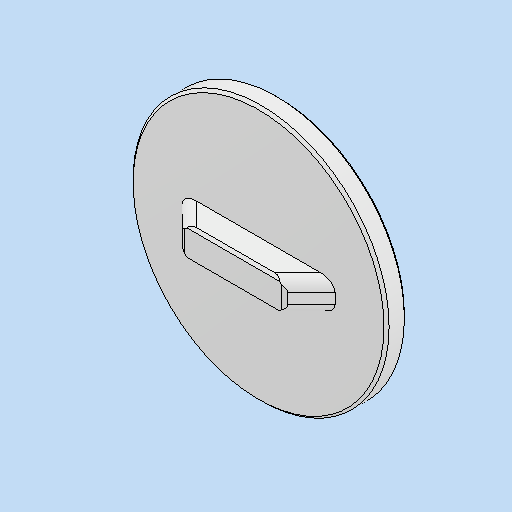
# Autodesk Inventor part: Sensor-Cap
Saved by Autodesk Inventor 2025 (Build 290162000, 162)
## iProperties
Created: 2025-02-18
Part Number: Sensor-Cap
Material: ABS Plastic
Document SubType Name: Modeling
Designer: kuzmin
Density: 1.06 g/cm^3
Appearance: Smooth - White
Author: kuzmin
Autodesk Inventor part; units mm, degrees
ref_plane "YZ Plane" through (0, 0, 0) normal (1, 0, 0) x (0, 1, 0)
ref_plane "XZ Plane" through (0, 0, 0) normal (0, 1, 0) x (-1, 0, 0)
ref_plane "XY Plane" through (0, 0, 0) normal (0, 0, 1) x (1, 0, 0)
sketch "Sketch1" plane through (0, 0, 0) normal (0, 0, 1) x (1, 0, 0)
  circle A0 centre (0, 0) radius 25.1
  dimension "d0" = 50.2
  constraints: 1 centre point, 1 coincident
  measures "d0" diameter of A0
extrude "Extrusion1" add sketch "Sketch1" along normal blind 4
sketch "Sketch2" plane through (0, 0, 4) normal (0, 0, 1) x (1, 0, 0)
  line L0 (-15, 3) -> (15, 3)
  line L1 (15, 3) -> (15, -3)
  line L2 (15, -3) -> (-15, -3)
  line L3 (-15, -3) -> (-15, 3)
  point P0 (0, 0)
  point P1 (15, 0)
  point P2 (0, 3)
  dimension "d3" = 30
  dimension "d4" = 6
  constraints: 8 end point, 2 midpoint, 2 parallel, 1 horizontal, 1 horizontal alignment, 1 perpendicular, 1 vertical alignment
  measures "d3" distance of L0.start L0.end
  measures "d4" distance of L0.end L1.end
extrude "Extrusion2" add sketch "Sketch2" along normal blind 5
chamfer "Chamfer1" distance 5 angle 45 2 edges at (15, 0, 9) (-15, 0, 9)
chamfer "Chamfer2" distance 0.5 angle 45 6 edges at (0, -3, 9) (-10.0001, 0, 9) (0, 3, 9) (10.0001, 0, 9) (-25.1, 0, 4) (-25.1, 0, 0)
fillet "Fillet2" radius 2 4 edges at (-12.7501, -3, 6.25) (-12.75, 3, 6.25) (12.75, -3, 6.25) (12.7501, 3, 6.2501)
body "Solid1"
